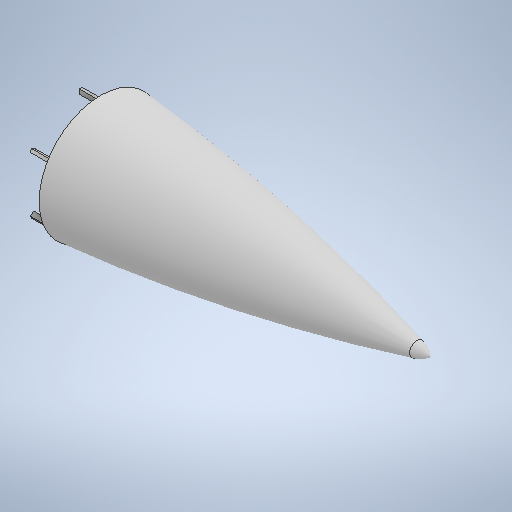
# Autodesk Inventor part: Nosecone(finale)tip
Saved by Autodesk Inventor 2025 (Build 290162000, 162)
## iProperties
Created: 2024-06-04
Part Number: Nosecone(finale)tip
Material: Generic
Document SubType Name: Sheet Metal
Designer: agnes
Density: 1 g/cm^3
Sheet Metal Rule: Default_mm
Appearance: Default
Author: agnes
Autodesk Inventor part; units mm, degrees
ref_plane "YZ Plane" through (0, 0, 0) normal (1, 0, 0) x (0, 1, 0)
ref_plane "XZ Plane" through (0, 0, 0) normal (0, 1, 0) x (-1, 0, 0)
ref_plane "XY Plane" through (0, 0, 0) normal (0, 0, 1) x (1, 0, 0)
sketch "Sketch1" plane through (0, 0, 0) normal (0, 0, 1) x (1, 0, 0)
  line L0 (0, 0) -> (286, 0)
  arc A0 (271.0494, 3.9199) -> (0, 50) centre (-140.2784, -1595.3524) ccw
  arc A1 (273.6055, 6.3591) -> (0, 53.0109) centre (-140.2784, -1595.3524) ccw
  arc A2 (286, 0) -> (273.6055, 6.3591) centre (265.6617, -24.3829) ccw
  arc A3 (280.1558, 0) -> (271.0494, 3.9199) centre (263.3021, -26.6152) ccw
  line L1 (-3, 0) -> (0, 0)
  line L2 (0, 50) -> (0, 53.0109)
  dimension "d0" = 286
  dimension "d1" = 50
  dimension "d2" = 3
  constraints: 8 point on circle, 6 end point, 4 centre point, 2 horizontal, 1 point on line, 1 tangent, 1 vertical
  measures "d0" distance of L0.start L0.end
  measures "d1" distance of L0.start L2.start
  measures "d2" radial gap between concentric circles of A0 A1
revolve "Revolution1" add sketch "Sketch1" angle 360 about axis through (0, 0, 0) along (1, 0, 0)
sketch "Sketch2" plane through (0, 0, 0) normal (-1, 0, 0) x (0, 0, 1)
  circle A0 centre (0, 0) radius 50 projected
  line L0 (0, 50) -> (2, 50)
  line L1 (2, 50) -> (2, 41)
  line L2 (2, 41) -> (0, 41)
  line L3 (0, 50) -> (-2, 50)
  line L4 (-2, 50) -> (-2, 41)
  line L5 (-2, 41) -> (0, 41)
  line L6 (-43.3013, 25) -> (-42.3013, 26.7321)
  line L7 (-42.3013, 26.7321) -> (-34.507, 22.2321)
  line L8 (-34.507, 22.2321) -> (-35.507, 20.5)
  line L9 (-43.3013, 25) -> (-44.3013, 23.2679)
  line L10 (-44.3013, 23.2679) -> (-36.507, 18.7679)
  line L11 (-36.507, 18.7679) -> (-35.507, 20.5)
  line L12 (-43.3013, -25) -> (-44.3013, -23.2679)
  line L13 (-44.3013, -23.2679) -> (-36.507, -18.7679)
  line L14 (-36.507, -18.7679) -> (-35.507, -20.5)
  line L15 (-43.3013, -25) -> (-42.3013, -26.7321)
  line L16 (-42.3013, -26.7321) -> (-34.507, -22.2321)
  line L17 (-34.507, -22.2321) -> (-35.507, -20.5)
  line L18 (0, -50) -> (-2, -50)
  line L19 (-2, -50) -> (-2, -41)
  line L20 (-2, -41) -> (0, -41)
  line L21 (0, -50) -> (2, -50)
  line L22 (2, -50) -> (2, -41)
  line L23 (2, -41) -> (0, -41)
  line L24 (43.3013, -25) -> (42.3013, -26.7321)
  line L25 (42.3013, -26.7321) -> (34.507, -22.2321)
  line L26 (34.507, -22.2321) -> (35.507, -20.5)
  line L27 (43.3013, -25) -> (44.3013, -23.2679)
  line L28 (44.3013, -23.2679) -> (36.507, -18.7679)
  line L29 (36.507, -18.7679) -> (35.507, -20.5)
  line L30 (43.3013, 25) -> (44.3013, 23.2679)
  line L31 (44.3013, 23.2679) -> (36.507, 18.7679)
  line L32 (36.507, 18.7679) -> (35.507, 20.5)
  line L33 (43.3013, 25) -> (42.3013, 26.7321)
  line L34 (42.3013, 26.7321) -> (34.507, 22.2321)
  line L35 (34.507, 22.2321) -> (35.507, 20.5)
  point P0 (-44.2666, -23.2479)
  point P1 (-42.2666, -26.712)
  point P2 (0, -41)
  point P3 (-2, -49.96)
  point P4 (2, -49.96)
  point P5 (42.2666, -26.712)
  point P6 (44.2666, -23.2479)
  point P7 (-42.2666, 26.712)
  point P8 (-44.2666, 23.2479)
  point P9 (44.2666, 23.2479)
  point P10 (42.2666, 26.712)
  point P11 (2, 49.96)
  point P12 (-2, 49.96)
  dimension "d4" = 2
  dimension "d5" = 9
  dimension "d6" = 2
  dimension "d9" = 360
  constraints: 72 end point, 6 point on line, 2 horizontal, 2 parallel, 2 perpendicular, 81 other
  measures "d4" distance of L1.end L2.end
  measures "d5" distance of L0.end L1.end
  measures "d6" distance of L5.end L4.end
extrude "Extrusion1" add sketch "Sketch2" against normal up to next contours L31 L32 L35 L34 A0 | A0 L25 L26 L29 L28 | L1 L2 L5 L4 A0 | A0 L19 L20 L23 L22 | L7 L8 L11 L10 A0 | A0 L13 L14 L17 L16
sketch "Sketch4" plane through (0, 0, 0) normal (-1, 0, 0) x (0, 0, 1)
  circle A0 centre (0, 0) radius 3.9199 projected
  circle A1 centre (0, 0) radius 50
  line L0 (0, 50) -> (1.25, 50)
  line L1 (1.25, 50) -> (1.25, 46)
  line L2 (1.25, 46) -> (0, 46)
  line L3 (0, 50) -> (-1.25, 50)
  line L4 (-1.25, 50) -> (-1.25, 46)
  line L5 (-1.25, 46) -> (0, 46)
  line L6 (-43.3013, 25) -> (-42.6763, 26.0825)
  line L7 (-42.6763, 26.0825) -> (-39.2122, 24.0825)
  line L8 (-39.2122, 24.0825) -> (-39.8372, 23)
  line L9 (-43.3013, 25) -> (-43.9263, 23.9175)
  line L10 (-43.9263, 23.9175) -> (-40.4622, 21.9175)
  line L11 (-40.4622, 21.9175) -> (-39.8372, 23)
  line L12 (-43.3013, -25) -> (-43.9263, -23.9175)
  line L13 (-43.9263, -23.9175) -> (-40.4622, -21.9175)
  line L14 (-40.4622, -21.9175) -> (-39.8372, -23)
  line L15 (-43.3013, -25) -> (-42.6763, -26.0825)
  line L16 (-42.6763, -26.0825) -> (-39.2122, -24.0825)
  line L17 (-39.2122, -24.0825) -> (-39.8372, -23)
  line L18 (0, -50) -> (-1.25, -50)
  line L19 (-1.25, -50) -> (-1.25, -46)
  line L20 (-1.25, -46) -> (0, -46)
  line L21 (0, -50) -> (1.25, -50)
  line L22 (1.25, -50) -> (1.25, -46)
  line L23 (1.25, -46) -> (0, -46)
  line L24 (43.3013, -25) -> (42.6763, -26.0825)
  line L25 (42.6763, -26.0825) -> (39.2122, -24.0825)
  line L26 (39.2122, -24.0825) -> (39.8372, -23)
  line L27 (43.3013, -25) -> (43.9263, -23.9175)
  line L28 (43.9263, -23.9175) -> (40.4622, -21.9175)
  line L29 (40.4622, -21.9175) -> (39.8372, -23)
  line L30 (43.3013, 25) -> (43.9263, 23.9175)
  line L31 (43.9263, 23.9175) -> (40.4622, 21.9175)
  line L32 (40.4622, 21.9175) -> (39.8372, 23)
  line L33 (43.3013, 25) -> (42.6763, 26.0825)
  line L34 (42.6763, 26.0825) -> (39.2122, 24.0825)
  line L35 (39.2122, 24.0825) -> (39.8372, 23)
  point P0 (-42.6627, 26.0747)
  point P1 (-43.9127, 23.9097)
  point P2 (-43.9127, -23.9097)
  point P3 (-42.6627, -26.0747)
  point P4 (0, -46)
  point P5 (-1.25, -49.9844)
  point P6 (1.25, -49.9844)
  point P7 (42.6627, -26.0747)
  point P8 (43.9127, -23.9097)
  point P9 (43.9127, 23.9097)
  point P10 (42.6627, 26.0747)
  point P11 (1.25, 49.9844)
  point P12 (-1.25, 49.9844)
  dimension "d29" = 1.25
  dimension "d30" = 4
  dimension "d31" = 1.25
  dimension "d34" = 360
  constraints: 72 end point, 6 point on line, 2 horizontal, 2 parallel, 2 perpendicular, 1 coincident, 82 other
  measures "d29" distance of L1.end L2.end
  measures "d30" distance of L0.end L1.end
  measures "d31" distance of L5.end L4.end
extrude "Extrusion3" add sketch "Sketch4" along normal blind 17 contours L31 L32 L35 L34 A1 | A1 L25 L26 L29 L28 | L1 L2 L5 L4 A1 | A1 L19 L20 L23 L22 | L7 L8 L11 L10 A1 | A1 L13 L14 L17 L16
equation "\"BendRadius\" = Thickness"
equation "\"BendReliefWidth\" = Thickness"
equation "\"BendReliefDepth\" = 0.5 * Thickness"
equation "\"CornerReliefSize\" = 4 * Thickness"
equation "\"MinimumRemnant\" = 2 * Thickness"
equation "\"TransitionRadius\" = BendRadius"
equation "\"JacobiRadiusSize\" = BendRadius"
equation "\"GapSize\" = Thickness"
equation "\"Thickness\" = 0.5"
body "Solid1"
